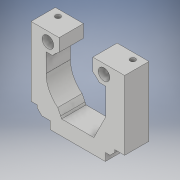
# Autodesk Inventor part: 30_CUBE_openSIM_Rodholder
Saved by Autodesk Inventor 2019 (Build 230136000, 136)
## iProperties
Created: 2020-08-19
Part Number: 30_CUBE_openSIM_Rodholder
Material: Generic
Document SubType Name: Modeling
Designer: wanghaoran
Density: 1 g/cm^3
Appearance: Default
Author: wanghaoran
Autodesk Inventor part; units mm, degrees
ref_plane "YZ Plane" through (0, 0, 0) normal (1, 0, 0) x (0, 1, 0)
ref_plane "XZ Plane" through (0, 0, 0) normal (0, 1, 0) x (-1, 0, 0)
ref_plane "XY Plane" through (0, 0, 0) normal (0, 0, 1) x (1, 0, 0)
sketch "Sketch1" plane through (0, 0, 0) normal (0, 0, 1) x (1, 0, 0)
  line L0 (0, 0) -> (50, 0)
  line L1 (50, 0) -> (50, 36.921)
  line L2 (50, 36.921) -> (0, 36.921)
  line L3 (0, 36.921) -> (0, 0)
  dimension "d0" = 36.921
  dimension "d1" = 50
  constraints: 8 end point, 2 parallel, 1 horizontal, 1 perpendicular
  measures "d0" distance of L0.end L1.end
  measures "d1" distance of L1.end L2.end
extrude "Extrusion1" add sketch "Sketch1" along normal blind 13
sketch "Sketch4" plane through (0, 0, 0) normal (0, 0, -1) x (-1, 0, 0)
  line L0 (-10, -8) -> (-40, -8)
  line L1 (-45.066, 0) -> (-2.934, 0)
  line L2 (-10.3, -8) -> (-10.3, -3.845)
  line L3 (-10.3, -3.845) -> (-5.7813, -3.845)
  line L4 (-5.7813, -3.845) -> (-3.234, -1.2977)
  line L5 (-3.234, -1.2977) -> (-3.234, 0)
  line L6 (-44.766, 0) -> (-44.766, -1.2977)
  line L7 (-44.766, -1.2977) -> (-42.2187, -3.845)
  line L8 (-42.2187, -3.845) -> (-39.7, -3.845)
  line L9 (-39.7, -3.845) -> (-39.7, -8)
  line L10 (0, 0) -> (-2.934, 0)
  line L11 (0, 0) -> (-50, 0) projected
  point P0 (-45.066, -1.422)
  dimension "d27" = 2.934
  constraints: 22 end point, 5 point on line
  measures "d27" distance of L10.start L10.end
extrude "Extrusion4" add sketch "Sketch4" against normal blind 13
sketch "Sketch2" plane through (0, 0, 0) normal (0, -1, 0) x (1, 0, 0)
  circle A0 centre (44.9, 3.5) radius 1.4
  circle A1 centre (4.9, 3.5) radius 1.4
  line L0 (50, 0) -> (50, 13) projected
  circle A2 centre (45.7, 9) radius 2.5
  circle A3 centre (4.1, 9) radius 2.5
  line L1 (0, 0) -> (0, 13) projected
  line L2 (0, 13) -> (50, 13) projected
  dimension "d4" = 2.8
  dimension "d5" = 2.8
  dimension "d7" = 40
  dimension "d8" = 5
  dimension "d9" = 5
  dimension "d10" = 5.5
  dimension "d13" = 4.1
  dimension "d14" = 5.5
  dimension "d15" = 4
  dimension "d16" = 4.9
  dimension "d17" = 41.6
  dimension "d20" = 4
  constraints: 4 centre point
  measures "d4" diameter of A0
  measures "d5" diameter of A1
  measures "d7" distance of A1.centre A0.centre
  measures "d8" diameter of A2
  measures "d9" diameter of A3
  measures "d10" vertical distance of A0.centre A2.centre
  measures "d13" distance from line of L1 A3.centre
  measures "d14" vertical distance of A1.centre A3.centre
  measures "d15" distance from line of L2 A3.centre
  measures "d16" distance from line of L1 A1.centre
  measures "d17" distance of A3.centre A2.centre
  measures "d20" distance from line of L2 A2.centre
extrude "Extrusion2" cut sketch "Sketch2" along normal blind 10 and the other way blind 5
sketch "Sketch7" plane through (0, 0, 0) normal (0, 0, -1) x (-1, 0, 0)
  arc A0 (17, 30.1329) -> (13.5279, 26.921) centre (26, 16.921) ccw
  line L0 (10, 26.921) -> (13.5279, 26.921)
  line L1 (10, 12.8998) -> (10, 26.921)
  line L2 (15.8642, 1.1093) -> (10, 12.8998)
  line L3 (16.416, 0) -> (33.6258, 0)
  line L4 (16.416, 0) -> (15.8642, 1.1093)
  line L5 (34.1776, 1.1093) -> (33.6258, 0)
  line L6 (35.7354, 4.2414) -> (34.1776, 1.1093)
  arc A1 (35.7354, 4.2414) -> (41.9856, 16.8076) centre (26, 16.921) ccw
  line L7 (42, 26.921) -> (42, 16.8366)
  line L8 (38.4721, 26.921) -> (42, 26.921)
  arc A2 (38.4721, 26.921) -> (35, 30.1328) centre (26, 16.921) ccw
  line L9 (35, 36.921) -> (35, 30.1328)
  line L10 (17, 30.1329) -> (17, 36.921)
  circle A3 centre (11, 31.921) radius 3.1
  circle A4 centre (41, 31.921) radius 3.1
  line L11 (42, 16.8366) -> (41.9856, 16.8076)
  line L12 (17, 36.921) -> (35, 36.921)
  line L13 (17, 35.9386) -> (35, 35.9386)
  line L14 (35, 35.9386) -> (35, 37.4386)
  line L15 (35, 37.4386) -> (17, 37.4386)
  line L16 (17, 37.4386) -> (17, 35.9386)
  line L17 (0, 36.921) -> (0, 0) projected
  line L18 (0, 36.921) -> (-15, 36.921)
  line L19 (0, 36.921) -> (15, 36.921) construction
  line L20 (-33, 35.9386) -> (-15, 35.9386)
  line L21 (-33, 36.921) -> (-15, 36.921)
  line L22 (-15, 37.4386) -> (-33, 37.4386)
  line L23 (-33, 37.4386) -> (-33, 35.9386)
  line L24 (-33, 30.1329) -> (-33, 36.921)
  arc A5 (-33, 30.1329) -> (-36.4721, 26.921) centre (-24, 16.921) ccw
  circle A6 centre (-39, 31.921) radius 3.1
  line L25 (-40, 26.921) -> (-36.4721, 26.921)
  line L26 (-40, 12.8998) -> (-40, 26.921)
  line L27 (-34.1358, 1.1093) -> (-40, 12.8998)
  line L28 (-33.584, 0) -> (-16.3742, 0)
  line L29 (-33.584, 0) -> (-34.1358, 1.1093)
  line L30 (-8, 16.8366) -> (-8.0144, 16.8076)
  arc A7 (-14.2646, 4.2414) -> (-8.0144, 16.8076) centre (-24, 16.921) ccw
  line L31 (-14.2646, 4.2414) -> (-15.8224, 1.1093)
  line L32 (-15.8224, 1.1093) -> (-16.3742, 0)
  line L33 (-8, 26.921) -> (-8, 16.8366)
  line L34 (-15, 35.9386) -> (-15, 37.4386)
  arc A8 (-11.5279, 26.921) -> (-15, 30.1328) centre (-24, 16.921) ccw
  line L35 (-11.5279, 26.921) -> (-8, 26.921)
  circle A9 centre (-9, 31.921) radius 3.1
  line L36 (-15, 36.921) -> (-15, 30.1328)
  point P0 (-35, 36.921)
  dimension "d33" = 1.5
  dimension "d34" = 15
  dimension "d35" = 180
  dimension "d39" = 1.5
  constraints: 72 end point, 12 point on circle, 10 centre point, 4 horizontal, 4 parallel, 4 point on line, 2 perpendicular, 1 collinear
  measures "d33" distance of L15.start L13.end
  measures "d34" distance of L17.start L18.end
  measures "d35" angle of L18 L19
  measures "d39" distance of L22.start L20.end
extrude "Extrusion7" cut sketch "Sketch7" against normal blind 13 contours L23 L21 L34 L20 | L20 L36 A8 L35 L33 L30 A7 L31 L32 L28 L29 L27 L26 L25 A5 L24 | L23 L22 L34 L21 | A6 | A9
sketch "Sketch8" plane through (0, 36.921, 13) normal (0, 1, 0) x (1, 0, 0)
  circle A0 centre (4.9, 9.5) radius 1.4 projected
  circle A1 centre (44.9, 9.5) radius 1.4 projected
  point P0 (0, 13)
extrude "Extrusion8" cut sketch "Sketch8" against normal blind 10
body "Solid1"
